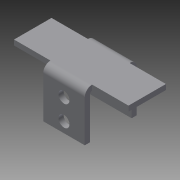
# Autodesk Inventor part: Winch mount frange
Saved by Autodesk Inventor 2013 (Build 170138000, 138)
## iProperties
Created: 2013-02-03
Part Number: Winch mount frange
Material: Generic
Document SubType Name: Sheet Metal
Designer: Arpan
Density: 1 g/cm^3
Sheet Metal Rule: Default
Author: Arpan
Autodesk Inventor part; units mm, degrees
ref_plane "YZ Plane" through (0, 0, 0) normal (1, 0, 0) x (0, 1, 0)
ref_plane "XZ Plane" through (0, 0, 0) normal (0, 1, 0) x (-1, 0, 0)
ref_plane "XY Plane" through (0, 0, 0) normal (0, 0, 1) x (1, 0, 0)
sketch "Sketch5" plane through (-25.4, 29.845, -1.27) normal (0, 1, 0) x (1, 0, 0)
  line L0 (25.4, 22.86) -> (25.4, 0)
  line L1 (0, 0) -> (0, 22.86)
  line L2 (0, 22.86) -> (-22.225, 22.86)
  line L3 (-22.225, 22.86) -> (-22.225, 0)
  line L4 (-22.225, 0) -> (0, 0)
  line L5 (25.4, 0) -> (47.625, 0)
  line L6 (47.625, 0) -> (47.625, 22.86)
  line L7 (47.625, 22.86) -> (25.4, 22.86)
  point P0 (25.4, -1.27)
  dimension "d30" = 22.225
  dimension "d31" = 22.86
  dimension "d32" = 22.225
  measures "d30" distance of L1.end L2.end
  measures "d31" distance of L2.end L3.end
  measures "d32" distance of L0.end L5.end
sketch "Sketch1" plane through (0, 0, 0) normal (0, 0, 1) x (1, 0, 0)
  line L0 (0, 0) -> (-25.4, 0)
  line L1 (-25.4, 0) -> (-25.4, 25.4)
  line L2 (-25.4, 25.4) -> (0, 25.4)
  line L3 (0, 25.4) -> (0, 0)
  dimension "d0" = 25.4
  dimension "d1" = 25.4
  measures "d0" distance of L0.start L0.end
  measures "d1" distance of L0.end L1.end
extrude "Plate1" add sketch "Sketch1" along normal blind 3.175
sketch "Sketch2" plane through (0, 26.67, -1.27) normal (0, 1, 0) x (-1, 0, 0)
  line L0 (25.4, 0) -> (0, 0)
  line L1 (0, 0) -> (0, -22.86)
  line L2 (0, -22.86) -> (25.4, -22.86)
  line L3 (25.4, -22.86) -> (25.4, 0)
  constraints: 6 end point, 1 horizontal, 1 perpendicular, 1 vertical
edge flange "Flange1" height 27.305 angle 90 thickness 3.175 bend radius 1.27 thickness toward (0, 1, 0) relief tear relief width 3.175 relief depth 1.5875 edges at (-12.7, 25.4, 0) wall of the first edge with corners at (-25.4, 26.67, -1.27) (0, 26.67, -1.27) (0, 26.67, -24.13) (-25.4, 26.67, -24.13)
bend "Bend1"
corner "Corner1"
sketch "Sketch3" plane through (0, 0, 3.175) normal (0, 0, 1) x (1, 0, 0)
  line L0 (-25.4, 25.4) -> (0, 25.4) projected
  line L1 (-25.4, 25.4) -> (-12.7, 25.4)
  line L2 (-12.7, 25.4) -> (-12.7, 19.05)
  line L3 (-12.7, 19.05) -> (-12.7, 12.7)
  line L4 (-12.7, 12.7) -> (-12.7, 6.35)
  circle A0 centre (-12.7, 19.05) radius 3.3782
  circle A1 centre (-12.7, 6.35) radius 3.3782
  dimension "d13" = 6.35
  dimension "d14" = 6.35
  dimension "d15" = 6.35
  dimension "d16" = 6.7564
  dimension "d17" = 6.7564
  constraints: 8 end point, 2 centre point, 2 coincident, 2 collinear, 1 midpoint, 1 perpendicular
  measures "d13" distance of L1.end L2.end
  measures "d14" distance of L2.end L3.end
  measures "d15" distance of L3.end L4.end
  measures "d16" diameter of A0
  measures "d17" diameter of A1
sketch "Sketch4" plane through (0, 25.4, -25.4) normal (0, 0, -1) x (-1, 0, 0)
  line L0 (25.4, 0) -> (0, 0)
  line L1 (0, 0) -> (0, -25.4)
  line L2 (0, -25.4) -> (25.4, -25.4)
  line L3 (25.4, -25.4) -> (25.4, 0)
  constraints: 6 end point, 1 horizontal, 1 perpendicular, 1 vertical
edge flange "Flange2" height 29.845 angle 90 thickness 3.175 bend radius 1.27 thickness toward (0, 0, -1) relief tear relief width 3.175 relief depth 1.5875 edges at (-12.7, 26.67, -24.13) wall of the first edge with corners at (-25.4, 25.4, -25.4) (0, 25.4, -25.4) (0, 0, -25.4) (-25.4, 0, -25.4)
bend "Bend2"
corner "Corner2"
extrude "Extrusion1" cut sketch "Sketch3" against normal blind 38.1
sheet face with bend "Face2" sketch "Sketch5" thickness 3.175 toward (0, -1, 0) bend radius 1.27 relief tear relief width 3.175 relief depth 1.5875
bend "Bend3"
equation "\"d3\" = BendReliefWidth"
equation "\"d4\" = BendReliefDepth"
equation "\"d5\" = MinimumRemnant"
equation "\"d6\" = BendRadius"
equation "\"d10\" = CornerReliefSize"
equation "\"d11\" = GapSize"
equation "\"d12\" = JacobiRadiusSize"
equation "\"d18\" = BendReliefWidth"
equation "\"d19\" = BendReliefDepth"
equation "\"d20\" = MinimumRemnant"
equation "\"d21\" = BendRadius"
equation "\"d25\" = CornerReliefSize"
equation "\"d26\" = GapSize"
equation "\"d27\" = JacobiRadiusSize"
equation "\"d34\" = BendReliefWidth"
equation "\"d36\" = MinimumRemnant"
equation "\"d35\" = BendReliefDepth"
equation "\"d37\" = BendRadius"
equation "\"BendRadius\" = Thickness"
equation "\"BendReliefWidth\" = Thickness"
equation "\"BendReliefDepth\" = 0.5 * Thickness"
equation "\"CornerReliefSize\" = 4 * Thickness"
equation "\"MinimumRemnant\" = 2 * Thickness"
equation "\"TransitionRadius\" = BendRadius"
equation "\"JacobiRadiusSize\" = Thickness"
equation "\"GapSize\" = Thickness"
equation "\"d2\" = BendRadius"
equation "\"Thickness\" = 3.175"
body "Solid1"
